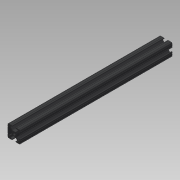
# Autodesk Inventor part: 1003
Saved by Autodesk Inventor 2013 (Build 170138000, 138)
## iProperties
Company: 80/20 Inc.
Created: 2013-09-06
Part Number: 1003
Material: Generic
Document SubType Name: Modeling
Density: 1 g/cm^3
Catalog Web Link: 8020.net
Vendor: 80/20 Inc.
Engineer: Ross Bowman
Author: Ross Bowman
Keywords: T-Slot, Extrusion, 80/20, 8020, Quick Frame, HT
Autodesk Inventor part; units mm, degrees
ref_plane "YZ Plane" through (0, 0, 0) normal (1, 0, 0) x (0, 1, 0)
ref_plane "XZ Plane" through (0, 0, 0) normal (0, 1, 0) x (-1, 0, 0)
ref_plane "XY Plane" through (0, 0, 0) normal (0, 0, 1) x (1, 0, 0)
sketch "Sketch1" plane through (0, 0, 0) normal (0, 0, 1) x (1, 0, 0)
  circle A0 centre (0, 0) radius 2.6035
  arc A1 (-8.7683, 7.1606) -> (-10.4902, 6.4464) centre (-9.4812, 6.4464) ccw
  line L0 (-5.4405, 3.8388) -> (-8.7683, 7.1606)
  arc A2 (-4.5085, 1.5917) -> (-5.4405, 3.8388) centre (-7.6835, 1.5917) ccw
  line L1 (-4.5085, -1.5917) -> (-4.5085, 1.5917)
  arc A3 (-5.4405, -3.8388) -> (-4.5085, -1.5917) centre (-7.6835, -1.5917) ccw
  line L2 (-8.7534, -7.1457) -> (-5.4405, -3.8388)
  arc A4 (-10.4902, -6.4254) -> (-8.7534, -7.1457) centre (-9.4724, -6.4254) ccw
  line L3 (-10.4902, 6.4464) -> (-10.4902, -6.4254)
  arc A5 (-7.1342, -8.7551) -> (-6.4164, -10.4902) centre (-6.4164, -9.4742) ccw
  line L4 (-7.1342, -8.7551) -> (-3.7967, -5.4237)
  arc A6 (-1.5536, -4.4958) -> (-3.7967, -5.4237) centre (-1.5536, -7.6708) ccw
  line L5 (-1.5536, -4.4958) -> (1.5536, -4.4958)
  arc A7 (3.7967, -5.4237) -> (1.5536, -4.4958) centre (1.5536, -7.6708) ccw
  line L6 (3.7967, -5.4237) -> (7.1285, -8.7494)
  arc A8 (6.4083, -10.4902) -> (7.1285, -8.7494) centre (6.4083, -9.4709) ccw
  line L7 (6.4083, -10.4902) -> (4.2875, -10.4902)
  arc A9 (4.2875, -10.4902) -> (3.2385, -11.5392) centre (4.2875, -11.5392) ccw
  line L8 (3.2385, -11.5392) -> (3.2385, -11.651)
  arc A10 (3.2385, -11.651) -> (4.2875, -12.7) centre (4.2875, -11.651) ccw
  line L9 (4.2875, -12.7) -> (5.3171, -12.7)
  arc A11 (6.3331, -12.7) -> (5.3171, -12.7) centre (5.8251, -12.7) ccw
  line L10 (6.3331, -12.7) -> (9.5504, -12.7)
  arc A12 (10.5664, -12.6998) -> (9.5504, -12.7) centre (10.0584, -12.7) ccw
  arc A13 (10.5664, -12.6998) -> (12.6998, -10.5664) centre (10.5918, -10.5918) ccw
  arc A14 (12.7, -9.5504) -> (12.6998, -10.5664) centre (12.7, -10.0584) ccw
  line L11 (12.7, -9.5504) -> (12.7, -6.3331)
  arc A15 (12.7, -5.3171) -> (12.7, -6.3331) centre (12.7, -5.8251) ccw
  line L12 (12.7, -5.3171) -> (12.7, -4.2875)
  arc A16 (12.7, -4.2875) -> (11.651, -3.2385) centre (11.651, -4.2875) ccw
  line L13 (11.651, -3.2385) -> (11.5392, -3.2385)
  arc A17 (11.5392, -3.2385) -> (10.4902, -4.2875) centre (11.5392, -4.2875) ccw
  line L14 (10.4902, -4.2875) -> (10.4902, -6.4021)
  arc A18 (8.737, -7.1292) -> (10.4902, -6.4021) centre (9.4628, -6.4021) ccw
  line L15 (8.737, -7.1292) -> (5.4405, -3.8388)
  arc A19 (4.5085, -1.5917) -> (5.4405, -3.8388) centre (7.6835, -1.5917) ccw
  line L16 (4.5085, -1.5917) -> (4.5085, 1.5917)
  arc A20 (5.4405, 3.8388) -> (4.5085, 1.5917) centre (7.6835, 1.5917) ccw
  line L17 (5.4405, 3.8388) -> (8.737, 7.1292)
  arc A21 (10.4902, 6.4021) -> (8.737, 7.1292) centre (9.4628, 6.4021) ccw
  line L18 (10.4902, 6.4021) -> (10.4902, 4.2875)
  arc A22 (10.4902, 4.2875) -> (11.5392, 3.2385) centre (11.5392, 4.2875) ccw
  line L19 (11.5392, 3.2385) -> (11.651, 3.2385)
  arc A23 (11.651, 3.2385) -> (12.7, 4.2875) centre (11.651, 4.2875) ccw
  line L20 (12.7, 4.2875) -> (12.7, 5.3171)
  arc A24 (12.7, 6.3331) -> (12.7, 5.3171) centre (12.7, 5.8251) ccw
  line L21 (12.7, 6.3331) -> (12.7, 9.5504)
  arc A25 (12.6998, 10.5664) -> (12.7, 9.5504) centre (12.7, 10.0584) ccw
  arc A26 (12.6998, 10.5664) -> (10.5664, 12.6998) centre (10.5918, 10.5918) ccw
  arc A27 (9.5504, 12.7) -> (10.5664, 12.6998) centre (10.0584, 12.7) ccw
  line L22 (9.5504, 12.7) -> (6.3331, 12.7)
  arc A28 (5.3171, 12.7) -> (6.3331, 12.7) centre (5.8251, 12.7) ccw
  line L23 (5.3171, 12.7) -> (4.2875, 12.7)
  arc A29 (4.2875, 12.7) -> (3.2384, 11.651) centre (4.2875, 11.651) ccw
  line L24 (3.2384, 11.651) -> (3.2384, 11.5392)
  arc A30 (3.2384, 11.5392) -> (4.2875, 10.4902) centre (4.2875, 11.5392) ccw
  line L25 (4.2875, 10.4902) -> (6.4768, 10.4902)
  arc A31 (7.2072, 8.7245) -> (6.4768, 10.4902) centre (6.4768, 9.4563) ccw
  line L26 (7.2072, 8.7245) -> (3.9003, 5.4237)
  arc A32 (1.6573, 4.4958) -> (3.9003, 5.4237) centre (1.6573, 7.6708) ccw
  line L27 (1.6573, 4.4958) -> (-1.5536, 4.4958)
  arc A33 (-3.7966, 5.4237) -> (-1.5536, 4.4958) centre (-1.5536, 7.6708) ccw
  line L28 (-3.7966, 5.4237) -> (-7.1341, 8.7551)
  arc A34 (-6.4164, 10.4902) -> (-7.1341, 8.7551) centre (-6.4164, 9.4742) ccw
  line L29 (-6.4164, 10.4902) -> (-4.2875, 10.4902)
  arc A35 (-4.2875, 10.4902) -> (-3.2384, 11.5392) centre (-4.2875, 11.5392) ccw
  line L30 (-3.2384, 11.5392) -> (-3.2384, 11.651)
  arc A36 (-3.2384, 11.651) -> (-4.2875, 12.7) centre (-4.2875, 11.651) ccw
  line L31 (-4.2875, 12.7) -> (-5.3171, 12.7)
  arc A37 (-6.3331, 12.7) -> (-5.3171, 12.7) centre (-5.8251, 12.7) ccw
  line L32 (-6.3331, 12.7) -> (-9.5504, 12.7)
  arc A38 (-10.5664, 12.6998) -> (-9.5504, 12.7) centre (-10.0584, 12.7) ccw
  arc A39 (-10.5664, 12.6998) -> (-12.6998, 10.5664) centre (-10.5918, 10.5918) ccw
  arc A40 (-12.7, 9.5504) -> (-12.6998, 10.5664) centre (-12.7, 10.0584) ccw
  line L33 (-12.7, 9.5504) -> (-12.7, 6.3331)
  arc A41 (-12.7, 5.3171) -> (-12.7, 6.3331) centre (-12.7, 5.8251) ccw
  line L34 (-12.7, 5.3171) -> (-12.7, -5.3171)
  arc A42 (-12.7, -6.3331) -> (-12.7, -5.3171) centre (-12.7, -5.8251) ccw
  line L35 (-12.7, -6.3331) -> (-12.7, -9.5504)
  arc A43 (-12.6998, -10.5664) -> (-12.7, -9.5504) centre (-12.7, -10.0584) ccw
  arc A44 (-12.6998, -10.5664) -> (-10.5664, -12.6998) centre (-10.5918, -10.5918) ccw
  arc A45 (-9.5504, -12.7) -> (-10.5664, -12.6998) centre (-10.0584, -12.7) ccw
  line L36 (-9.5504, -12.7) -> (-6.3331, -12.7)
  arc A46 (-5.3171, -12.7) -> (-6.3331, -12.7) centre (-5.8251, -12.7) ccw
  line L37 (-5.3171, -12.7) -> (-4.2875, -12.7)
  arc A47 (-4.2875, -12.7) -> (-3.2385, -11.651) centre (-4.2875, -11.651) ccw
  line L38 (-3.2385, -11.651) -> (-3.2385, -11.5392)
  arc A48 (-3.2385, -11.5392) -> (-4.2875, -10.4902) centre (-4.2875, -11.5392) ccw
  line L39 (-4.2875, -10.4902) -> (-6.4164, -10.4902)
  constraints: 96 point on circle, 80 end point, 49 centre point
extrude "Extrusion1" add sketch "Sketch1" against normal blind 304.8
body "Solid1"
